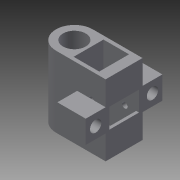
# Autodesk Inventor part: XEndTop
Saved by Autodesk Inventor 2015 (Build 190159000, 159)
## iProperties
Created: 2014-08-09
Part Number: XEndTop
Material: Generic
Document SubType Name: Modeling
Designer: Jack
Density: 1 g/cm^3
Appearance: Default
Author: Jack
Autodesk Inventor part; units mm, degrees
ref_plane "YZ Plane" through (0, 0, 0) normal (1, 0, 0) x (0, 1, 0)
ref_plane "XZ Plane" through (0, 0, 0) normal (0, 1, 0) x (-1, 0, 0)
ref_plane "XY Plane" through (0, 0, 0) normal (0, 0, 1) x (1, 0, 0)
sketch "Sketch1" plane through (0, 0, 0) normal (0, 0, 1) x (1, 0, 0)
  circle A0 centre (0, 0) radius 8
  circle A1 centre (0, 0) radius 13
  line L0 (0, 13) -> (35, 13)
  line L1 (35, 13) -> (35, -13)
  line L2 (35, -13) -> (0, -13)
  dimension "d0" = 16
  dimension "d1" = 26
  dimension "d2" = 48
  constraints: 6 end point, 2 centre point, 2 coincident, 2 horizontal, 2 point on circle, 2 tangent, 1 perpendicular
  measures "d0" diameter of A0
  measures "d1" diameter of A1
extrude "Extrusion1" add sketch "Sketch1" against normal blind 50
sketch "Sketch2" plane through (0, 0, 0) normal (0, 0, 1) x (1, 0, 0)
  circle A0 centre (0, 0) radius 8 projected
  line L0 (35, 13) -> (0, 13) projected
  line L1 (10, 10.5) -> (28, 10.5)
  line L2 (28, 10.5) -> (28, -10.5)
  line L3 (28, -10.5) -> (10, -10.5)
  line L4 (10, -10.5) -> (10, 10.5)
  dimension "d5" = 18
  dimension "d6" = 21
  dimension "d7" = 10
  dimension "d8" = 2.5
  constraints: 8 end point, 2 parallel, 1 horizontal, 1 perpendicular
  measures "d5" distance of L1.start L1.end
  measures "d6" distance of L3.end L1.start
  measures "d7" distance from line of A0.centre L4
  measures "d8" distance between parallel lines of L0 L1
extrude "Extrusion2" cut sketch "Sketch2" against normal up to surface (50 mm away) contours L1 L2 L3 L4
sketch "Sketch3" plane through (0, 13, 0) normal (0, 1, 0) x (1, 0, 0)
  line L0 (0, 50) -> (35, 50) projected
  line L1 (0, 0) -> (0, 50) projected
  circle A0 centre (25, 32.5) radius 2
  circle A1 centre (25, 17.5) radius 2
  line L2 (-8, 50) -> (8, 50) projected
  line L3 (8, 0) -> (-8, 0) projected
  dimension "d11" = 4
  dimension "d12" = 4
  dimension "d13" = 15
  dimension "d14" = 25
  dimension "d15" = 17.5
  constraints: 2 centre point, 1 vertical alignment
  measures "d11" diameter of A0
  measures "d12" diameter of A1
  measures "d13" distance of A0.centre A1.centre
  measures "d14" distance from line of L1 A0.centre
  measures "d15" distance from line of L0 A0.centre
extrude "Extrusion3" cut sketch "Sketch3" along normal blind 50 and the other way blind 29.25
sketch "Sketch4" plane through (35, -13, 0) normal (1, 0, 0) x (0, 0, -1)
  line L0 (0, 0) -> (0, 26) projected
  line L1 (0, 0) -> (50, 0) projected
  line L2 (18, 2.5) -> (32, 2.5)
  line L3 (32, 2.5) -> (32, 23.5)
  line L4 (32, 23.5) -> (18, 23.5)
  line L5 (18, 23.5) -> (18, 2.5)
  point P0 (0, 13)
  dimension "d20" = 14
  dimension "d21" = 21
  dimension "d22" = 18
  dimension "d23" = 2.5
  constraints: 8 end point, 2 parallel, 1 horizontal, 1 perpendicular
  measures "d20" distance of L3.end L4.end
  measures "d21" distance of L4.end L2.start
  measures "d22" distance between parallel lines of L0 L5
  measures "d23" distance between parallel lines of L1 L2
extrude "Extrusion4" cut sketch "Sketch4" against normal up to surface (7 mm away)
chamfer "Chamfer1" distance 5 angle 45 2 edges at (28, 0, -32) (28, 0, -18)
sketch "Sketch5" plane through (35, -13, 0) normal (1, 0, 0) x (0, 0, -1)
  line L0 (0, 0) -> (50, 0) projected
  line L1 (50, 26) -> (50, 0) projected
  line L2 (0, 26) -> (50, 26) projected
  circle A0 centre (25, 33) radius 4
  circle A1 centre (25, -7) radius 4
  line L3 (0, 26) -> (50, 26) projected
  line L4 (17, 26) -> (17, 40)
  line L5 (17, 40) -> (33, 40)
  line L6 (33, 40) -> (33, 26)
  line L7 (0, 0) -> (50, 0) projected
  line L8 (17, 0) -> (17, -14)
  line L9 (17, -14) -> (33, -14)
  line L10 (33, -14) -> (33, 0)
  point P0 (0, 13)
  dimension "d29" = 8
  dimension "d30" = 8
  dimension "d31" = 25
  dimension "d32" = 40
  dimension "d33" = 7
  dimension "d34" = 14
  dimension "d35" = 14
  dimension "d36" = 8
  dimension "d37" = 8
  constraints: 12 end point, 6 perpendicular, 4 point on line, 3 vertical alignment, 2 centre point
  measures "d29" diameter of A0
  measures "d30" diameter of A1
  measures "d31" distance from line of L1 A0.centre
  measures "d32" distance of A0.centre A1.centre
  measures "d33" distance from line of L2 A0.centre
  measures "d34" distance between parallel lines of L2 L5
  measures "d35" distance between parallel lines of L0 L9
  measures "d36" distance from line of A1.centre L10
  measures "d37" distance from line of L8 A1.centre
extrude "Extrusion5" add sketch "Sketch5" against normal blind 22
body "Solid1"
